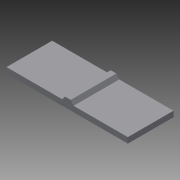
# Autodesk Inventor part: Sketch - Ball Shifting Shaft
Saved by Autodesk Inventor 2013 (Build 170138000, 138)
## iProperties
Created: 2013-06-06
Part Number: Sketch - Ball Shifting Shaft
Material: Generic
Document SubType Name: Modeling
Designer: mvarma
Density: 1 g/cm^3
Author: mvarma
Autodesk Inventor part; units mm, degrees
ref_plane "YZ Plane" through (0, 0, 0) normal (1, 0, 0) x (0, 1, 0)
ref_plane "XZ Plane" through (0, 0, 0) normal (0, 1, 0) x (-1, 0, 0)
ref_plane "XY Plane" through (0, 0, 0) normal (0, 0, 1) x (1, 0, 0)
sketch "Sketch1" plane through (0, 0, 0) normal (0, 0, 1) x (1, 0, 0)
  line L0 (0, 0) -> (4.7625, 0)
  line L1 (4.7625, 3.1115) -> (3.9687, 3.1115) construction
  line L2 (0, 3.1115) -> (0, 0)
  line L3 (4.7625, 0) -> (12.7, 0)
  line L4 (12.7, 0) -> (12.7, 3.1115) construction
  line L5 (12.7, 5.1753) -> (11.1125, 5.1753) construction
  line L6 (4.7625, 5.1753) -> (4.7625, 3.1115) construction
  line L7 (2.3812, 3.1115) -> (2.3812, 0) construction
  line L8 (8.7312, 5.1753) -> (8.7312, 0) construction
  line L9 (2.3812, 3.1115) -> (2.3812, 5.4927) construction
  circle A0 centre (2.3812, 5.4927) radius 2.3812 construction
  line L10 (6.35, 5.1753) -> (6.35, 0) construction
  line L11 (11.1125, 5.1753) -> (11.1125, 0) construction
  line L12 (4.7625, 3.1115) -> (12.7, 3.1115) construction
  line L13 (6.35, 5.1753) -> (4.7625, 5.1753) construction
  line L14 (4.7625, 3.1115) -> (4.7625, 0) construction
  line L15 (11.1125, 5.1753) -> (10.3187, 5.1753) construction
  line L16 (12.7, 3.1115) -> (12.7, 5.1753) construction
  line L17 (8.7312, 5.1753) -> (8.7312, 7.5565) construction
  circle A1 centre (8.7312, 7.5565) radius 2.3813 construction
  line L18 (0.7937, 3.1115) -> (0.7937, 0)
  line L19 (3.9687, 3.1115) -> (3.9687, 0)
  line L20 (7.1437, 5.1753) -> (7.1437, 0)
  line L21 (10.3187, 5.1753) -> (10.3187, 0)
  line L22 (3.9687, 3.1115) -> (0.7937, 3.1115)
  line L23 (0.7937, 3.1115) -> (0, 3.1115)
  line L24 (10.3187, 5.1753) -> (8.7312, 5.1753)
  line L25 (7.1437, 5.1753) -> (6.35, 5.1753) construction
  line L26 (8.7312, 5.1753) -> (7.1437, 5.1753)
  line L27 (3.9687, 3.1115) -> (7.1437, 5.1753)
  line L28 (0, 0) -> (0, 5.5563) construction
  line L29 (0, 5.5563) -> (17.4625, 5.5563) construction
  line L30 (0, 5.5563) -> (0, 7.9375) construction
  line L31 (0, 7.9375) -> (17.4625, 7.9375) construction
  line L32 (12.7, 3.1115) -> (13.4937, 3.1115) construction
  line L33 (12.7, 0) -> (17.4625, 0)
  line L34 (17.4625, 0) -> (17.4625, 3.1115)
  line L35 (15.0812, 0) -> (15.0812, 3.1115) construction
  line L36 (13.4937, 3.1115) -> (13.4937, 0)
  line L37 (16.6687, 3.1115) -> (16.6687, 0)
  line L38 (13.4937, 3.1115) -> (15.0812, 3.1115)
  line L39 (16.6687, 3.1115) -> (17.4625, 3.1115)
  line L40 (15.0812, 3.1115) -> (16.6687, 3.1115)
  line L41 (15.0812, 3.1115) -> (15.0812, 5.4928) construction
  line L42 (10.3187, 5.1753) -> (13.4937, 3.1115)
  line L43 (0, -12.7) -> (0, 0) construction
  line L44 (0, -7.1437) -> (26.1938, -7.1437) construction
  line L45 (0, -4.7625) -> (26.1938, -4.7625) construction
  line L46 (26.1938, -4.7625) -> (26.1938, -7.1437) construction
  line L47 (26.1938, -7.1437) -> (26.1938, -12.7) construction
  line L48 (26.1938, -12.7) -> (0, -12.7) construction
  line L49 (26.1938, -6.35) -> (34.3852, -6.35) construction
  line L50 (26.1938, -12.7) -> (34.3852, -12.7) construction
  line L51 (34.3852, -12.7) -> (34.3852, -6.35) construction
  line L52 (16.6688, -4.7625) -> (16.6688, -12.7) construction
  circle A2 centre (16.6688, -5.1435) radius 2.3813 construction
  circle A3 centre (16.6688, -7.2073) radius 2.3813 construction
  circle A4 centre (10.3187, -5.1435) radius 2.3813 construction
  circle A5 centre (10.3187, -7.2073) radius 2.3813 construction
  line L53 (10.3187, -4.7625) -> (10.3187, -12.7) construction
  line L54 (0, -7.5248) -> (26.1938, -7.5248) construction
  line L55 (8.7312, -7.5248) -> (8.7312, -12.7) construction
  line L56 (5.5562, -7.5248) -> (5.5562, -12.7) construction
  line L57 (18.2563, -7.5248) -> (18.2563, -12.7) construction
  line L58 (21.4313, -7.5248) -> (21.4313, -12.7) construction
  line L59 (0, -9.5885) -> (26.1938, -9.5885) construction
  line L60 (5.5562, -9.5885) -> (8.7312, -7.5248) construction
  line L61 (18.2563, -7.5248) -> (21.4312, -9.5885) construction
  line L62 (11.9062, -7.5248) -> (11.9062, -12.7) construction
  line L63 (15.0812, -7.5248) -> (15.0812, -12.7) construction
  line L64 (11.9062, -7.5248) -> (15.0812, -9.5885) construction
  line L65 (21.4313, -9.3266) -> (34.3852, -9.3266) construction
  line L66 (24.6063, -9.3266) -> (24.6063, -12.7) construction
  line L67 (21.4313, -9.3266) -> (20.1197, -7.1437) construction
  line L68 (26.1938, -9.5885) -> (30.9563, -9.5885) construction
  line L69 (30.9563, -9.5885) -> (30.9563, -12.7) construction
  line L70 (31.75, -9.3266) -> (31.75, -12.7) construction
  line L71 (31.75, -12.7) -> (29.723, -9.3266) construction
  line L72 (0, -4.7625) -> (-1.5875, -4.7625) construction
  line L73 (-1.5875, -4.7625) -> (-1.5875, -9.3266) construction
  line L74 (-1.5875, -9.3266) -> (5.5562, -9.3266) construction
  line L75 (1.4233, 7.874) -> (3.7622, 7.874)
  line L76 (5.5562, 3.1115) -> (7.1437, 5.1753)
  line L77 (10.3187, 5.1753) -> (11.9062, 3.1115)
  line L78 (11.9062, 3.1115) -> (13.4937, 3.1115)
  line L79 (5.5562, 3.1115) -> (3.9687, 3.1115)
  dimension "d8" = 6.35
  dimension "d9" = 5.1753
  dimension "d10" = 4.7625
  dimension "d11" = 2.3813
  dimension "d12" = 3.175
  dimension "d13" = 3.175
  dimension "d14" = 4.7625
  dimension "d15" = 2.3813
  dimension "d16" = 3.1115
  dimension "d17" = 5.5563
  dimension "d18" = 7.9375
  dimension "d19" = 6.35
  dimension "d20" = 3.175
  dimension "d21" = 2.3813
  dimension "d25" = 12.7
  dimension "d26" = 5.5563
  dimension "d27" = 7.9375
  dimension "d28" = 26.1938
  dimension "d29" = 8.1915
  dimension "d30" = 6.35
  dimension "d33" = 9.525
  dimension "d35" = 0.381
  dimension "d36" = 0.0635
  dimension "d38" = 6.35
  dimension "d39" = 0.381
  dimension "d40" = 0.381
  dimension "d41" = 0.0635
  dimension "d42" = 0.0635
  dimension "d43" = 9.525
  dimension "d46" = 1.5875
  dimension "d47" = 4.7625
  dimension "d48" = 1.5875
  dimension "d49" = 4.7625
  dimension "d50" = 3.1115
  dimension "d51" = 1.5875
  dimension "d52" = 4.7625
  dimension "d53" = 3.3734
  dimension "d54" = 3.175
  dimension "d55" = 31
  dimension "d56" = 9.525
  dimension "d57" = 9.525
  dimension "d59" = 0.7937
  dimension "d60" = 31
  dimension "d61" = 1.5875
  dimension "d62" = 3.3734
  dimension "d63" = 0.0635
  dimension "d70" = 0.7937
  dimension "d71" = 0.7937
  constraints: 158 end point, 51 point on line, 31 perpendicular, 26 parallel, 9 vertical, 6 coincident, 5 horizontal, 4 centre point, 4 midpoint, 3 collinear, 3 equal radius, 2 tangent, 2 vertical alignment, 25 other
  measures "d8" distance between parallel lines of L8 L7
  measures "d9" distance of L3.end L5.start
  measures "d10" distance between parallel lines of L11 L10
  measures "d11" distance of L8.start L17.end
  measures "d12" distance between parallel lines of L19 L18
  measures "d13" distance between parallel lines of L21 L20
  measures "d14" distance between parallel lines of L2 L14
  measures "d15" distance of L7.start L9.end
  measures "d16" distance between parallel lines of L0 L22
  measures "d17" distance of L0.start L28.end
  measures "d18" distance of L0.start L30.end
  measures "d19" distance between parallel lines of L35 L8
  measures "d20" distance between parallel lines of L37 L36
  measures "d21" distance of L35.end L41.end
  measures "d25" distance of L43.start L0.start
  measures "d26" distance from line of L44 L43.start
  measures "d27" distance from line of L43.start L45
  measures "d28" distance of L45.start L45.end
  measures "d29" distance of L49.start L49.end
  measures "d30" distance of L50.end L49.end
  measures "d33" distance between parallel lines of L46 L52
  measures "d35" distance from line of L31 L17.end
  measures "d36" distance from line of L29 point (15.081, 5.493)
  measures "d38" distance between parallel lines of L52 L53
  measures "d39" distance from line of L45 A4.centre
  measures "d40" distance from line of L45 A2.centre
  measures "d41" distance from line of L44 A3.centre
  measures "d42" distance from line of L44 A5.centre
  measures "d43" distance between parallel lines of L19 L36
  measures "d46" distance between parallel lines of L55 L53
  measures "d47" distance between parallel lines of L56 L53
  measures "d48" distance between parallel lines of L52 L57
  measures "d49" distance between parallel lines of L58 L52
  measures "d51" distance between parallel lines of L53 L62
  measures "d52" distance between parallel lines of L53 L63
  measures "d53" distance between parallel lines of L50 L65
  measures "d54" distance between parallel lines of L58 L66
  measures "d55" angle of L58 L67
  measures "d56" distance from line of L66 L64.end
  measures "d57" distance from line of L69 L61.end
  measures "d59" distance between parallel lines of L70 L69
  measures "d60" angle of L70 L71
  measures "d61" distance of L45.start L72.end
  measures "d63" distance between parallel lines of L31 L75
  measures "d70" distance from line of L4 L77.end
  measures "d71" distance from line of L14 L76.start
extrude "Extrusion1" add sketch "Sketch1" along normal blind 25.4 contours L2 L23 L18 L0 | L18 L22 L19 L0 | L19 L79 L76 L20 L3 L0 | L20 L26 L24 L21 L3 | L21 L77 L78 L36 L33 L3 | L36 L38 L40 L37 L33
sketch "Sketch2" plane through (16.6687, 0, 0) normal (1, 0, 0) x (0, 0, -1)
  line L0 (0, 0) -> (0, 3.1115) projected
  line L1 (0, 3.1115) -> (-25.4, 3.1115) projected
  line L2 (-25.4, 0) -> (-25.4, 3.1115) projected
  line L3 (0, 0) -> (-25.4, 0) projected
extrude "Extrusion2" add sketch "Sketch2" along normal blind 25.4
sketch "Sketch3" plane through (0, 0, 0) normal (-1, 0, 0) x (0, 0, 1)
  line L0 (0, 3.1115) -> (0, 0) projected
  line L1 (0, 0) -> (25.4, 0) projected
  line L2 (25.4, 3.1115) -> (25.4, 0) projected
  line L3 (0, 3.1115) -> (25.4, 3.1115) projected
extrude "Extrusion3" add sketch "Sketch3" along normal blind 25.4
fillet "Fillet1" radius 2.54 4 edges at (10.3187, 5.1753, 12.7) (7.1437, 5.1753, 12.7) (11.9062, 3.1115, 12.7) (5.5562, 3.1115, 12.7)
equation "\"d19\" = d8"
equation "\"d26\" = d17"
equation "\"d27\" = d18"
equation "\"d39\" = d35"
equation "\"d40\" = d39"
equation "\"d41\" = d36"
equation "\"d42\" = d41"
equation "\"d50\" = d16"
equation "\"d51\" = d46"
equation "\"d52\" = d47"
equation "\"d57\" = d56"
equation "\"d60\" = d55"
equation "\"d62\" = d53"
body "Solid1"
